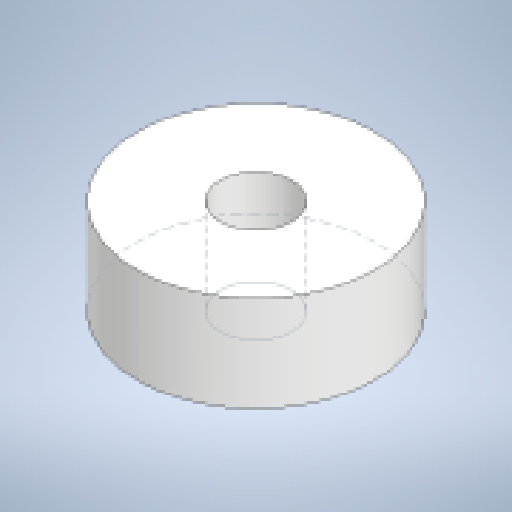
# Autodesk Inventor part: bearing 3-10x4
Saved by Autodesk Inventor 2025 (Build 290162000, 162)
## iProperties
Created: 2023-12-22
Part Number: bearing 3-10x4
Material: アセタール樹脂、白
Document SubType Name: Modeling
Designer: user
Density: 1.425 g/cm^3
Appearance: 滑らか - 白
Mass: 0.407386 g
Surface Area: 3.06305 cm^2
Volume: 0.285885 cm^3
Author: user
Autodesk Inventor part; units mm, degrees
ref_plane "YZ Plane" through (0, 0, 0) normal (1, 0, 0) x (0, 1, 0)
ref_plane "XZ Plane" through (0, 0, 0) normal (0, 1, 0) x (-1, 0, 0)
ref_plane "XY Plane" through (0, 0, 0) normal (0, 0, 1) x (1, 0, 0)
sketch "Sketch1" plane through (0, 0, 0) normal (0, 1, 0) x (-1, 0, 0)
  circle A0 centre (0, 0) radius 1.5
  circle A1 centre (0, 0) radius 5
  dimension "d0" = 3
  dimension "d1" = 10
  constraints: 2 centre point, 2 coincident
  measures "d0" diameter of A0
  measures "d1" diameter of A1
extrude "Extrusion1" add sketch "Sketch1" along normal blind 4
body "Solid1"
